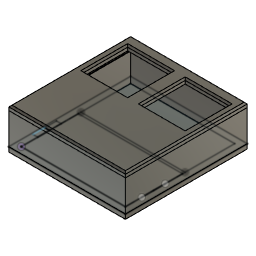
kaypad_nogap_V2 (Autodesk Fusion 360 design; units mm, degrees)
Autodesk Fusion 360 part; units mm, degrees
sketch "Sketch1" plane through (0, 0, 0) normal (0, 0, 1) x (1, 0, 0) in component "case"
  line L0 (0, 0) -> (33.3333, 0)
  line L1 (33.3333, 0) -> (33.3333, 35)
  line L2 (33.3333, 35) -> (0, 35)
  line L3 (0, 35) -> (0, 0)
  line L4 (-2, 37) -> (-2, -2)
  line L5 (-2, -2) -> (35.3333, -2)
  line L6 (35.3333, -2) -> (35.3333, 37)
  line L7 (35.3333, 37) -> (-2, 37)
  line L8 (33.3333, 0) -> (33.3333, 18.3) construction
  line L9 (33.3333, 18.3) -> (0, 18.3)
  line L10 (0, 18.3) -> (0, 0)
  line L11 (0, 0) -> (33.3333, 0)
  line L12 (33.3333, 0) -> (33.3333, 18.3)
  line L13 (33.3333, 19.1) -> (0, 19.1)
  line L14 (33.3333, 18.3) -> (33.3333, 9) construction
  line L15 (33.3333, 12.75) -> (33.3333, 9)
  line L16 (33.3333, 5.25) -> (33.3333, 9)
  line L17 (0, 18.3) -> (0, 9) construction
  line L18 (0, 9) -> (-1.5, 9)
  line L19 (-1.5, 9) -> (-1.5, 12.75)
  line L20 (-1.5, 12.75) -> (0, 12.75)
  line L21 (0, 12.75) -> (0, 9) construction
  line L22 (0, 9) -> (-1.5, 9)
  line L23 (-1.5, 9) -> (-1.5, 5.25)
  line L24 (-1.5, 5.25) -> (0, 5.25)
  line L25 (0, 5.25) -> (0, 9)
  dimension "d3" = 33.3333
  dimension "d4" = 35
  dimension "d5" = 2
  dimension "d6" = 18.3
  dimension "d7" = 0.8
  dimension "d16" = 9.3
  dimension "d23" = 9.3
  dimension "d24" = 1.5
  dimension "d25" = 3.75
  dimension "d26" = 3.75
  constraint horizontal L0
  constraint vertical L1
  constraint horizontal L2
  constraint vertical L3
  constraint coincident L0.start L3.end
  constraint perpendicular L5 L8
  constraint horizontal L9
  constraint vertical L10
  constraint horizontal L11
  constraint vertical L12
  constraint perpendicular L9 L14
  constraint vertical L15
  constraint vertical L16
  constraint perpendicular L9 L17
  constraint horizontal L18
  constraint vertical L19
  constraint horizontal L20
  constraint vertical L21
  constraint horizontal L22
  constraint vertical L23
  constraint horizontal L24
  constraint vertical L25
  measures "d3" distance of L0.start L0.end
  measures "d4" distance of L0.start L2.end
  measures "d6" distance of L0.end L8.end
  measures "d16" distance of L8.end L14.end
  measures "d23" distance of L9.end L17.end
  measures "d24" distance of L17.end L18.end
  measures "d25" distance of L17.end L20.end
  measures "d26" distance of L17.end L24.end
extrude "Extrude1" add sketch "Sketch1" against normal blind 2 contours L0 L1 L3 L9 L10 L11 L12 L15 L16 L25 | L3 L10 L18 L22 L23 L24 L25 | L3 L10 L18 L19 L20 L22 | L1 L3 L9 L13 | L1 L2 L3 L13 | L4 L5 L6 L7 makes body 1 in component "case"
ref_plane "WorkPlane1" through (16.6667, 9.15, 1.7) normal (0, 0, 1) x (1, 0, 0) in component "case"
extrude "Extrude2" add sketch "Sketch1" along normal blind 10 contours L3 L10 L18 L22 L23 L24 L25 | L3 L10 L18 L19 L20 L22 | L4 L5 L6 L7 bodies 1 in component "case"
extrude "Extrude3" add sketch "Sketch1" along normal blind 1.7 contours L1 L3 L9 L13 bodies 1 in component "case"
chamfer "Chamfer1" distance 0.5 angle 45 1 edges at (16.6667, 19.1, 0) on bodies 1 in component "case"
sketch "Sketch3" plane through (16.6667, 9.15, 1.7) normal (0, 0, 1) x (1, 0, 0)
  line L0 (-18.1667, 3.6) -> (-16.6667, 3.6)
  line L1 (-18.1667, -0.15) -> (-18.1667, 3.6)
  line L2 (-18.1667, -0.15) -> (-18.1667, -3.9)
  line L3 (-18.1667, -3.9) -> (-16.6667, -3.9)
  line L4 (-16.6667, 25.85) -> (-16.6667, -9.15)
  line L5 (-16.6667, 3.6) -> (-20, 3.6)
  line L6 (-20, 3.6) -> (-20, -3.9)
  line L7 (-20, -3.9) -> (-16.6667, -3.9)
  line L8 (-16.6667, -3.9) -> (-16.6667, 3.6)
  dimension "d31" = 7.5
  constraint horizontal L5
  constraint vertical L6
  constraint horizontal L7
  constraint vertical L8
  constraint coincident L0.end L5.start
  measures "d31" distance of L0.end L3.end
extrude "Extrude4" cut sketch "Sketch3" along normal blind 2.6 and the other way blind 0.1 bodies 1 in component "case"
chamfer "Chamfer2" distance 1 angle 45 2 edges at (-1, 12.75, 1.6) (-1, 5.25, 1.6) on bodies 1 in component "case"
sketch "Sketch4" plane through (-2, 0, 0) normal (-1, 0, 0) x (0, -1, 0)
  line L0 (-6.25, 1.6) -> (-11.75, 1.6)
  line L1 (-11.75, 1.6) -> (-12.75, 2.6)
  line L2 (-12.75, 2.6) -> (-12.75, 4.3)
  line L3 (-12.75, 4.3) -> (-5.25, 4.3)
  line L4 (-5.25, 4.3) -> (-5.25, 2.6)
  line L5 (-5.25, 2.6) -> (-6.25, 1.6)
  line L6 (-37, 10) -> (-37, -2)
  line L7 (-37, -2) -> (2, -2)
  line L8 (2, -2) -> (2, 10)
  line L9 (2, 10) -> (-37, 10)
  line L10 (-12.75, 4.3) -> (-5.25, 4.3)
  line L11 (-5.25, 4.3) -> (-5.25, 2.6)
  line L12 (-6.25, 1.6) -> (-5.25, 2.6)
  line L13 (-6.25, 1.6) -> (-11.75, 1.6)
  line L14 (-12.75, 2.6) -> (-11.75, 1.6)
  line L15 (-12.75, 2.6) -> (-12.75, 4.3)
  line L16 (-4.25, 2.1858) -> (-5.8358, 0.6)
  line L17 (-5.8358, 0.6) -> (-12.1642, 0.6)
  line L18 (-12.1642, 0.6) -> (-13.75, 2.1858)
  line L19 (-13.75, 2.1858) -> (-13.75, 5.3)
  line L20 (-13.75, 5.3) -> (-4.25, 5.3)
  line L21 (-4.25, 5.3) -> (-4.25, 2.1858)
  dimension "d33" = -1
  measures "d33" distance of L5
extrude "Extrude5" cut sketch "Sketch4" against normal blind 0.5 contours L16 L17 L18 L19 L20 L21 bodies 1 in component "case"
fillet "Fillet1" radius 0.5 12 edges at (-1.5, 13.75, 3.7429) (-2, 13.75, 3.7429) (-1.5, 9, 5.3) (-2, 9, 5.3) (-1.5, 4.25, 3.7429) (-2, 4.25, 3.7429) (-1.5, 5.0429, 1.3929) (-2, 5.0429, 1.3929) (-2, 9, 0.6) (-1.5, 9, 0.6) (-1.5, 12.9571, 1.3929) (-2, 12.9571, 1.3929) on bodies 1 in component "case"
sketch "Sketch5" plane through (0, 0, 10) normal (0, 0, 1) x (-1, 0, 0)
  line L0 (-33.3333, -35) -> (-33.3333, 0)
  line L1 (-33.3333, 0) -> (0, 0)
  line L2 (0, 0) -> (0, -35)
  line L3 (0, -35) -> (-33.3333, -35)
  line L4 (-35.3333, -37) -> (2, -37)
  line L5 (2, -37) -> (2, 2)
  line L6 (2, 2) -> (-35.3333, 2)
  line L7 (-35.3333, 2) -> (-35.3333, -37)
  line L8 (-33.3333, -35) -> (0, -35)
  line L9 (-33.3333, 0) -> (-33.3333, -35)
  line L10 (0, 0) -> (0, -35)
  line L11 (-33.3333, 0) -> (0, 0)
  line L12 (0.8, 0.8) -> (0.8, -35.8)
  line L13 (-34.1333, -35.8) -> (0.8, -35.8)
  line L14 (-34.1333, 0.8) -> (-34.1333, -35.8)
  line L15 (-34.1333, 0.8) -> (0.8, 0.8)
  dimension "d38" = -0.8
extrude "Extrude6" cut sketch "Sketch5" against normal blind 1 contours L12 L13 L14 L15 bodies 1 in component "case"
sketch "Sketch1 (2)" plane through (0, 0, 10) normal (0, 0, 1) x (-1, 0, 0) in component "Lid"
  line L0 (0.8, 0.8) -> (0.8, -35.8)
  line L1 (0.8, -35.8) -> (-34.1333, -35.8)
  line L2 (-34.1333, -35.8) -> (-34.1333, 0.8)
  line L3 (-34.1333, 0.8) -> (0.8, 0.8)
  line L4 (-35.3333, -37) -> (2, -37)
  line L5 (2, -37) -> (2, 2)
  line L6 (2, 2) -> (-35.3333, 2)
  line L7 (-35.3333, 2) -> (-35.3333, -37)
  line L8 (0.8, -35.8) -> (-34.1333, -35.8)
  line L9 (-34.1333, -35.8) -> (-34.1333, 0.8)
  line L10 (-34.1333, 0.8) -> (0.8, 0.8)
  line L11 (0.8, 0.8) -> (0.8, -35.8)
  line L12 (0.6, 0.6) -> (0.6, -35.6)
  line L13 (0.6, -35.6) -> (-33.9333, -35.6)
  line L14 (-33.9333, -35.6) -> (-33.9333, 0.6)
  line L15 (-33.9333, 0.6) -> (0.6, 0.6)
  line L16 (-33.3333, 0) -> (-33.3333, -35)
  line L17 (-33.3333, -35) -> (0, -35)
  line L18 (0, -35) -> (0, 0)
  line L19 (0, 0) -> (-33.3333, 0)
  dimension "d41" = 0.2
  constraint horizontal L8
  constraint vertical L9
  constraint horizontal L10
  constraint vertical L11
  constraint coincident L2.end L3.start
  constraint coincident L0.end L1.start
extrude "Extrude1'" add sketch "Sketch1 (2)" against normal blind 0.8 separate body contours L12 L13 L14 L15 makes body 2 in component "Lid"
sketch "Sketch2" plane through (0, 0, 10) normal (0, 0, 1) x (-1, 0, 0) in component "Lid"
  line L0 (-33.3333, 0) -> (0, 0)
  line L1 (0, 0) -> (0, -35)
  line L2 (0, -35) -> (-33.3333, -35)
  line L3 (-33.3333, -35) -> (-33.3333, 0)
  line L4 (-33.9333, 0.6) -> (-33.9333, -35.6)
  line L5 (-33.9333, -35.6) -> (0.6, -35.6)
  line L6 (0.6, -35.6) -> (0.6, 0.6)
  line L7 (0.6, 0.6) -> (-33.9333, 0.6)
  line L8 (-35.3333, -37) -> (2, -37)
  line L9 (-35.3333, 2) -> (-35.3333, -37)
  line L10 (0.8, 0.8) -> (0.8, -35.8)
  line L11 (0.8, -35.8) -> (-34.1333, -35.8)
  line L12 (-34.1333, -35.8) -> (-34.1333, 0.8)
  line L13 (-34.1333, 0.8) -> (0.8, 0.8)
  line L14 (-35.3333, -37) -> (2, -37)
  line L15 (2, -37) -> (2, 2)
  line L16 (2, 2) -> (-35.3333, 2)
  line L17 (-35.3333, 2) -> (-35.3333, -37)
extrude "Extrude2'" add sketch "Sketch2" along normal blind 1.5 contours L0 L1 L2 L3 | L4 L5 L6 L7 | L8 L9 L14 L15 L16 L17 | L10 L11 L12 L13 bodies 2 in component "Lid"
sketch "Sketch3 (2)" plane through (0, 0, 11.5) normal (0, 0, 1) x (-1, 0, 0) in component "Lid"
  line L0 (-35.3333, 2) -> (-35.3333, -37)
  line L1 (-35.3333, -37) -> (2, -37)
  line L2 (2, -37) -> (2, 2)
  line L3 (2, 2) -> (-35.3333, 2)
  line L4 (-34.1333, -35.8) -> (-34.1333, 0.8)
  line L5 (0.8, 0.8) -> (0.8, -35.8)
  line L6 (0.8, -35.8) -> (-34.1333, -35.8)
  line L7 (-34.1333, -35.8) -> (-34.1333, 0.8)
  line L8 (-34.1333, 0.8) -> (0.8, 0.8)
  line L9 (-35.3333, -37) -> (2, -37)
  line L10 (2, -37) -> (2, 2)
  line L11 (2, 2) -> (-35.3333, 2)
  line L12 (-35.3333, 2) -> (-35.3333, -37)
  line L13 (-34.1333, -30.5029) -> (-32.8833, -30.5029) construction
  line L14 (-31.8035, -35.8) -> (-31.8035, -33.6) construction
  line L15 (-32.8833, -33.6) -> (-18.8833, -33.6)
  line L16 (-18.8833, -33.6) -> (-18.8833, -19.6)
  line L17 (-18.8833, -19.6) -> (-32.8833, -19.6)
  line L18 (-32.8833, -19.6) -> (-32.8833, -33.6)
  line L19 (-3.5652, -35.8) -> (-3.5652, -33.6) construction
  line L20 (0.8, -29.5336) -> (-0.45, -29.5336) construction
  line L21 (-0.45, -33.6) -> (-14.45, -33.6)
  line L22 (-14.45, -33.6) -> (-14.45, -19.6)
  line L23 (-14.45, -19.6) -> (-0.45, -19.6)
  line L24 (-0.45, -19.6) -> (-0.45, -33.6)
  dimension "d46" = 1.25
  dimension "d47" = 2.2
  dimension "d48" = 14
  dimension "d49" = 14
  dimension "d50" = 2.2
  dimension "d51" = 1.25
  dimension "d52" = 14
  dimension "d53" = 14
  constraint horizontal L13
  constraint coincident L7 L13.start
  constraint coincident L6 L14.start
  constraint perpendicular L6 L14
  constraint horizontal L15
  constraint vertical L16
  constraint horizontal L17
  constraint vertical L18
  constraint coincident L6 L19.start
  constraint perpendicular L6 L19
  constraint coincident L5 L20.start
  constraint perpendicular L5 L20
  constraint horizontal L21
  constraint vertical L22
  constraint horizontal L23
  constraint vertical L24
  measures "d46" distance of L13.start L13.end
  measures "d47" distance of L14.start L14.end
  measures "d48" distance of L15.start L15.end
  measures "d49" distance of L15.start L17.end
  measures "d50" distance of L19.start L19.end
  measures "d51" distance of L20.start L20.end
  measures "d52" distance of L21.start L21.end
  measures "d53" distance of L21.start L23.end
extrude "Extrude3'" cut sketch "Sketch3 (2)" against normal blind 2 contours L15 L16 L17 L18 | L21 L22 L23 L24 bodies 2 in component "Lid"
chamfer "Chamfer1'" distance 0.5 angle 45 12 edges at (25.8833, 33.6, 11.5) (18.8833, 26.6, 11.5) (7.45, 33.6, 11.5) (14.45, 26.6, 11.5) (0.45, 26.6, 11.5) (7.45, 19.6, 11.5) (25.8833, 19.6, 11.5) (32.8833, 26.6, 11.5) (16.6667, -2, 11.5) (-2, 17.5, 11.5) (16.6667, 37, 11.5) (35.3333, 17.5, 11.5) on bodies 2 in component "Lid"
chamfer "Chamfer3" distance 0.5 angle 45 4 edges at (35.3333, 17.5, -2) (16.6667, -2, -2) (16.6667, 37, -2) (-2, 17.5, -2) on bodies 1 in component "case"
component "case" placed x (1, 0, 0) y (0, 1, 0) z (0, 0, 1) at (0, 0, 0)
component "Lid" placed x (1, 0, 0) y (0, 1, 0) z (0, 0, 1) at (0, 0, 0)
